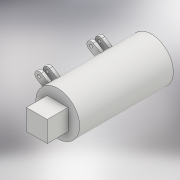
# Autodesk Inventor part: MockPitchMotor
Saved by Autodesk Inventor 2018 (Build 220112000, 112)
## iProperties
Created: 2018-03-27
Part Number: MockPitchMotor
Material: ABS Plastic
Document SubType Name: Modeling
Designer: mansu
Density: 1.06 g/cm^3
Appearance: Smooth - White
Author: mansu
Autodesk Inventor part; units mm, degrees
note: some values were not read from the file. Chosen so that the rebuilt part matches the saved one: pattern direction of "Rectangular Pattern2".
ref_plane "YZ Plane" through (0, 0, 0) normal (1, 0, 0) x (0, 1, 0)
ref_plane "XZ Plane" through (0, 0, 0) normal (0, 1, 0) x (-1, 0, 0)
sketch "Sketch1" plane through (0, 0, 0) normal (0, 1, 0) x (-1, 0, 0)
  circle A0 centre (0, 0) radius 21
  line L0 (10, 10) -> (-10, 10)
  line L1 (-10, 10) -> (-10, -10)
  line L2 (-10, -10) -> (10, -10)
  line L3 (10, -10) -> (10, 10)
  line L4 (10, 10) -> (-10, -10) construction
  line L5 (-10, 10) -> (10, -10) construction
  dimension "d0" = 42
  dimension "d1" = 20
  dimension "d2" = 20
  constraints: 12 end point, 2 midpoint, 2 parallel, 1 centre point, 1 coincident, 1 horizontal, 1 perpendicular
  measures "d0" diameter of A0
  measures "d1" distance of L2.end L1.end
  measures "d2" distance of L1.end L0.end
extrude "Extrusion1" add sketch "Sketch1" along normal blind 90 contours A0 | L3 L2 L1 L0
extrude "Extrusion2" add sketch "Sketch1" against normal blind 20 contours L3 L2 L1 L0
ref_plane "Work Plane1" through (0, 10, 0) normal (0, -1, 0) x (1, 0, 0)
sketch "Sketch2" plane through (0, 10, 0) normal (0, -1, 0) x (1, 0, 0)
  circle A0 centre (-25, 15) radius 1.5
  circle A1 centre (-25, -15) radius 1.5
  circle A2 centre (0, 0) radius 21 projected
  line L0 (-15.6197, 14.0366) -> (-22.942, 18.43)
  arc A3 (-22.942, 18.43) -> (-27.058, 11.57) centre (-25, 15) ccw
  line L1 (-27.058, 11.57) -> (-19.7357, 7.1766)
  line L2 (-19.7357, -7.1766) -> (-27.058, -11.57)
  arc A4 (-27.058, -11.57) -> (-22.942, -18.43) centre (-25, -15) ccw
  line L3 (-22.942, -18.43) -> (-15.6197, -14.0366)
  line L4 (-25, 15) -> (0, 0) construction
  line L5 (0, 0) -> (-25, -15) construction
  point P0 (-21, 0)
  dimension "d8" = 3
  dimension "d9" = 30
  dimension "d10" = 15
  dimension "d11" = 4
  dimension "d12" = 4
  dimension "d13" = 4
  constraints: 12 end point, 9 point on circle, 4 centre point, 4 parallel, 4 tangent, 2 concentric, 1 equal radius, 1 horizontal alignment, 1 vertical alignment
  measures "d8" diameter of A1
  measures "d9" distance of A1.centre A0.centre
  measures "d10" vertical distance of point (0, 0) A0.centre
  measures "d11" horizontal distance of A0.centre A2.start
  measures "d12" radius of A4
  measures "d13" radius of A3
extrude "Extrusion3" add sketch "Sketch2" along normal blind 3 contours A2 L1 A3 L0 | L3 A4 L2 A2
pattern_linear "Rectangular Pattern2" count 2 spacing 8 along (0, 1, 0) of "Extrusion3"
pattern_linear "Rectangular Pattern1" count 2 spacing 50 along (0, 1, 0) of "Extrusion3", "Rectangular Pattern2"
body "Solid1"
